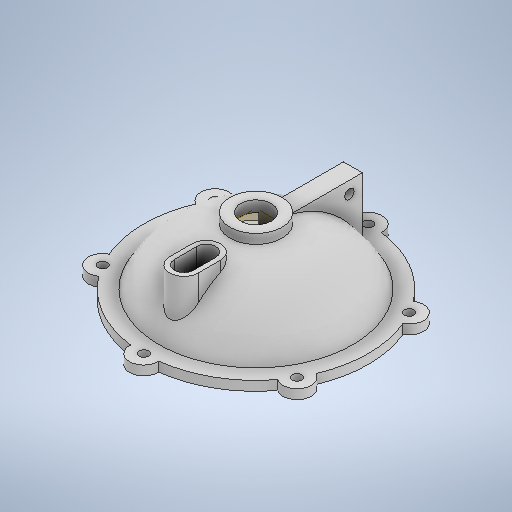
# Autodesk Inventor part: Bai_11
Saved by Autodesk Inventor 2025.1 (Build 291241000, 241)
## iProperties
Created: 2024-10-02
Part Number: Bai_11
Material: Generic
Document SubType Name: Modeling
Designer: msi
Density: 1 g/cm^3
Appearance: Default
Author: msi
Autodesk Inventor part; units mm, degrees
ref_plane "YZ Plane" through (0, 0, 0) normal (1, 0, 0) x (0, 1, 0)
ref_plane "XZ Plane" through (0, 0, 0) normal (0, 1, 0) x (-1, 0, 0)
ref_plane "XY Plane" through (0, 0, 0) normal (0, 0, 1) x (1, 0, 0)
sketch "Sketch1" plane through (0, 0, 0) normal (1, 0, 0) x (0, 1, 0)
  line L0 (0, 0) -> (64, 0)
  line L1 (0, 0) -> (56, 0)
  line L2 (0, 0) -> (8, 0)
  line L3 (0, 0) -> (0, -95)
  line L4 (0, 0) -> (0, -82)
  line L5 (0, 0) -> (6, 0)
  line L6 (64, 0) -> (64, -13)
  line L7 (64, -13) -> (64, -22)
  line L8 (56, 0) -> (56, -13) construction
  line L9 (56, -22) -> (64, -22) construction
  line L10 (56, -22) -> (56, -95) construction
  line L11 (56, -95) -> (0, -95) construction
  line L12 (64, -22) -> (56, -22)
  line L13 (0, -95) -> (0, -107)
  line L14 (0, -107) -> (8, -107)
  line L15 (8, -107) -> (8, -95)
  line L16 (113.6296, 0) -> (-73.0224, 0)
  line L17 (0, -82) -> (56, -82) construction
  line L18 (8, -95) -> (8, -82)
  line L19 (56, -82) -> (8, -82)
  line L20 (56, -82) -> (56, -22)
  line L21 (8, -95) -> (0, -95)
  arc A0 (0, -85.7011) -> (56, -22) centre (-35.8458, 2.2766) ccw construction
  line L22 (0, -82) -> (0, -85.7011)
  line L23 (56, -22) -> (56, -30)
  line L24 (56, -13) -> (56, 0) construction
  arc A1 (0, -82) -> (54.4542, -13) centre (-35.8458, 2.2766) ccw construction
  line L25 (64, -13) -> (54.4542, -13)
  line L26 (56, -22) -> (56, 0) construction
  arc A2 (8, -82) -> (56, -22) centre (-35.8458, 2.2766) ccw
  line L27 (-35.8458, 2.2766) -> (-35.8458, 0)
  arc A3 (0, -82) -> (54.4542, -13) centre (-35.8458, 2.2766) ccw
  line L28 (8, -82) -> (0, -82)
  point P0 (-35.8458, 1.1383)
  point P1 (8, -82)
  point P2 (8, -82)
  dimension "d0" = 64
  dimension "d1" = 56
  dimension "d2" = 8
  dimension "d3" = 95
  dimension "d4" = 82
  dimension "d5" = 6
  dimension "d6" = 13
  dimension "d7" = 9
  dimension "d12" = 12
  constraints: 58 end point, 12 point on line, 9 point on circle, 8 perpendicular, 8 vertical, 4 centre point, 4 collinear, 4 horizontal, 3 coincident, 1 midpoint, 1 other
  measures "d0" distance of L0.start L0.end
  measures "d1" distance of L0.start L1.end
  measures "d2" distance of L0.start L2.end
  measures "d3" distance of L0.start L3.end
  measures "d4" distance of L0.start L4.end
  measures "d5" distance of L0.start L5.end
  measures "d6" distance of L0.end L6.end
  measures "d7" distance of L6.end L7.end
  measures "d12" distance of L3.end L13.end
ref_plane "Work Plane3" through (0, 0, 0) normal (0, -1, 0) x (1, 0, 0)
sketch "Sketch3" plane through (0, 0, 0) normal (0, -1, 0) x (1, 0, 0)
  circle A0 centre (0, 0) radius 95 projected
  circle A1 centre (0, -95) radius 11.9643
  circle A2 centre (82.2724, -47.5) radius 11.9643
  circle A3 centre (82.2724, 47.5) radius 11.9643
  circle A4 centre (0, 95) radius 11.9643
  circle A5 centre (-82.2724, 47.5) radius 11.9643
  circle A6 centre (-82.2724, -47.5) radius 11.9643
  dimension "d15" = 360
  constraints: 6 centre point, 1 vertical alignment, 14 other
ref_plane "Work Plane1" through (0, 56, 0) normal (0, 1, 0) x (1, 0, 0)
extrude "Extrusion2" add sketch "Sketch3" against normal blind 8 contours A3 A0 | A0 A3 | A2 A0 | A0 A2 | A4 A0 | A0 A4 | A1 A0 | A0 A1 | A5 A0 | A0 A5 | A6 A0 | A0 A6
revolve "Revolution2" add sketch "Sketch1" angle 360 about axis through (0, 113.6296, 0) along (0, -1, 0) contours L0 L6 L25 A3 L3 | L28 L18 L21 L3 | A3 L25 L7 L12 A2 L28 | A2 L20 L19
sketch "Sketch5" plane through (0, 56, 0) normal (0, 1, 0) x (1, 0, 0)
  arc A0 (-75.6497, 57.4641) -> (-87.5902, 36.7825) centre (-82.2724, 47.5) ccw projected
  circle A1 centre (-82.2724, 47.5) radius 4
  circle A2 centre (-82.2724, -47.5) radius 4
  circle A3 centre (0, -95) radius 4
  circle A4 centre (82.2724, -47.5) radius 4
  circle A5 centre (82.2724, 47.5) radius 4
  circle A6 centre (0, 95) radius 4
  point P0 (0, 0)
  dimension "d20" = 8
  dimension "d23" = 360
  constraints: 6 centre point, 1 coincident, 13 other
  measures "d20" diameter of A1
extrude "Extrusion3" cut sketch "Sketch5" against normal blind 64
sketch "Sketch8" plane through (0, 64, 0) normal (0, 1, 0) x (1, 0, 0)
  circle A0 centre (0, 0) radius 13
  dimension "d39" = 26
  constraints: 1 centre point, 1 coincident
  measures "d39" diameter of A0
extrude "Extrusion4" cut sketch "Sketch8" against normal blind 64
sketch "Sketch9" plane through (0, 56, 0) normal (0, 1, 0) x (1, 0, 0)
  circle A0 centre (0, 0) radius 82 projected
  line L0 (0, 82) -> (67.9153, 82) construction
  line L1 (0, 82) -> (8, 82)
  line L2 (-82, 0) -> (82, 0)
  line L3 (8, 82) -> (8, 0)
  line L4 (8, 82) -> (-8, 82)
  line L5 (-8, 82) -> (-8, 0)
  line L6 (0, 0) -> (0, -42) construction
  line L7 (0, -42) -> (0, -61) construction
  circle A1 centre (0, -42) radius 12 construction
  circle A2 centre (0, -42) radius 8 construction
  circle A3 centre (0, -61) radius 12 construction
  circle A4 centre (0, -61) radius 8 construction
  line L8 (-12, -61) -> (-12, -42)
  line L9 (12, -61) -> (12, -42)
  line L10 (-12, -61) -> (12, -61) construction
  line L11 (-12, -42) -> (12, -42) construction
  arc A5 (-12, -61) -> (12, -61) centre (0, -61) ccw
  arc A6 (12, -42) -> (-12, -42) centre (0, -42) ccw
  arc A7 (8, -42) -> (-8, -42) centre (0, -42) ccw
  arc A8 (-8, -61) -> (8, -61) centre (0, -61) ccw
  line L12 (-8, -61) -> (-8, -42)
  line L13 (8, -61) -> (8, -42)
  point P0 (8, 81.6088)
  point P1 (-8, 81.6088)
  dimension "d42" = 8
  dimension "d43" = 16
  dimension "d44" = 42
  dimension "d45" = 19
  dimension "d46" = 24
  dimension "d47" = 16
  dimension "d48" = 24
  dimension "d49" = 16
  constraints: 28 end point, 20 point on circle, 8 centre point, 8 coincident, 8 point on line, 3 horizontal, 3 perpendicular, 3 vertical, 2 tangent, 1 parallel
  measures "d42" distance of L0.start L1.end
  measures "d43" distance of L1.end L4.end
  measures "d44" distance of L6.start L6.end
  measures "d45" distance of L6.end L7.end
  measures "d46" diameter of A1
  measures "d47" diameter of A2
  measures "d48" diameter of A3
  measures "d49" diameter of A4
extrude "Extrusion5" cut sketch "Sketch9" against normal blind 56 contours L2 A0 | A0 L5 L2 | L2 L3 A0
revolve "Revolution3" add sketch "Sketch1" angle 360 about axis through (0, 113.6296, 0) along (0, -1, 0) contours A3 L25 L7 L12 A2 L28
sketch "Sketch10" plane through (0, 56, 61) normal (0, 1, 0) x (1, 0, 0)
  circle A0 centre (0, 0) radius 8
  arc A1 (12, 19) -> (-12, 19) centre (0, 19) ccw projected
  circle A2 centre (0, 19) radius 8
  line L0 (-8, 0) -> (-8, 19)
  line L1 (8, 0) -> (8, 19)
  arc A3 (-12, 0) -> (12, 0) centre (0, 0) ccw projected
  line L2 (0, 0) -> (0, 19)
  line L3 (-8, 0) -> (8, 0)
  point P0 (0, 61)
  dimension "d54" = 16
  dimension "d55" = 16
  constraints: 8 end point, 4 point on circle, 2 centre point, 2 parallel, 2 vertical, 1 coincident, 1 horizontal, 1 tangent, 1 other
  measures "d54" diameter of A0
  measures "d55" diameter of A2
extrude "Extrusion6" cut sketch "Sketch10" against normal blind 56
sketch "Sketch11" plane through (8, 56, -20.4939) normal (1, 0, 0) x (0, 0, -1)
  point P0 (-20.4939, -56)
sketch "Sketch12" plane through (0, 56, 0) normal (0, 1, 0) x (1, 0, 0)
  arc A0 (8, 81.6088) -> (-8, 81.6088) centre (0, 0) ccw projected
  line L0 (0, 82) -> (-26.239, 82)
  line L1 (-26.239, 82) -> (20.0179, 82)
  line L2 (8, 81.6088) -> (8, 82)
  line L3 (-8, 81.6088) -> (-8, 82)
  circle A1 centre (0, 0) radius 82
  constraints: 8 end point, 3 point on line, 2 perpendicular, 1 coincident, 1 horizontal, 1 point on circle, 1 tangent, 1 vertical alignment, 2 other
extrude "Extrusion7" add sketch "Sketch12" against normal blind 56 contours A0 L1 L2 | A0 L3 L0
sketch "Sketch13" plane through (8, 56, -20.4939) normal (1, 0, 0) x (0, 0, -1)
  line L0 (61.4732, -0.0625) -> (61.5061, -10.0624)
  line L1 (61.5061, 0) -> (61.5061, -48) projected
  line L2 (61.5061, -10.0624) -> (50.5062, -10.0986)
  circle A0 centre (50.5062, -10.0986) radius 4
  point P0 (-20.4939, -56)
  dimension "d60" = 10
  dimension "d61" = 11
  dimension "d62" = 8
  constraints: 4 end point, 1 centre point, 1 coincident, 1 perpendicular, 1 point on line
  measures "d60" distance of L0.start L0.end
  measures "d61" distance of L0.end L2.end
  measures "d62" diameter of A0
extrude "Extrusion8" cut sketch "Sketch13" against normal blind 56
body "Solid1"
